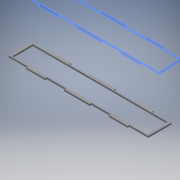
# Autodesk Inventor part: letreiro
Saved by Autodesk Inventor 2016 (Build 200138000, 138)
## iProperties
Created: 2017-06-07
Part Number: letreiro
Material: Generic
Document SubType Name: Modeling
Designer: fabio-note
Density: 1 g/cm^3
Appearance: Default
Author: fabio-note
Autodesk Inventor part; units mm, degrees
ref_plane "YZ Plane" through (0, 0, 0) normal (1, 0, 0) x (0, 1, 0)
ref_plane "XZ Plane" through (0, 0, 0) normal (0, 1, 0) x (-1, 0, 0)
ref_plane "XY Plane" through (0, 0, 0) normal (0, 0, 1) x (1, 0, 0)
sketch "Sketch1" plane through (0, 0, 0) normal (0, 0, 1) x (1, 0, 0)
  line L0 (-173, 32.5) -> (173, 32.5)
  line L1 (173, 32.5) -> (173, -32.5)
  line L2 (173, -32.5) -> (-173, -32.5)
  line L3 (-173, -32.5) -> (-173, 32.5)
  point P0 (0, 0)
  point P1 (173, 0)
  point P2 (0, 32.5)
  dimension "d0" = 65
  dimension "d1" = 346
  constraints: 8 end point, 2 midpoint, 2 parallel, 1 horizontal, 1 horizontal alignment, 1 perpendicular, 1 vertical alignment
  measures "d0" distance between parallel lines of L0 L2
  measures "d1" distance between parallel lines of L3 L1
extrude "Extrusion1" add sketch "Sketch1" along normal blind 4
sketch "Sketch2" plane through (0, 0, 4) normal (0, 0, 1) x (1, 0, 0)
  line L0 (-159, 25.5) -> (159, 25.5)
  line L1 (159, 25.5) -> (159, -25.5)
  line L2 (159, -25.5) -> (-159, -25.5)
  line L3 (-159, -25.5) -> (-159, 25.5)
  line L4 (173, 32.5) -> (-173, 32.5) projected
  line L5 (-173, 32.5) -> (-173, -32.5) projected
  line L6 (-173, -32.5) -> (173, -32.5) projected
  line L7 (173, -32.5) -> (173, 32.5) projected
  point P0 (0, 0)
  dimension "d4" = 7
  dimension "d5" = 14
  dimension "d6" = 7
  dimension "d7" = 14
  constraints: 8 end point, 2 parallel, 1 horizontal, 1 perpendicular
  measures "d4" distance between parallel lines of L4 L0
  measures "d5" distance between parallel lines of L5 L3
  measures "d6" distance between parallel lines of L6 L2
  measures "d7" distance between parallel lines of L7 L1
extrude "Extrusion2" cut sketch "Sketch2" against normal blind 10 contours L0 L1 L2 L3
sketch "Esboço3" plane through (0, 0, 4) normal (0, 0, 1) x (1, 0, 0)
  line L0 (-118.5, 32.5) -> (-118.5, 28.5)
  line L1 (-118.5, 28.5) -> (-165, 28.5)
  line L2 (-70.5, 32.5) -> (-24, 32.5)
  line L3 (-24, 32.5) -> (-24, 28.5)
  line L4 (-24, 28.5) -> (-70.5, 28.5)
  line L5 (-70.5, 28.5) -> (-70.5, 32.5)
  circle A0 centre (-118.5, 28.5) radius 1
  circle A1 centre (-70.5, 28.5) radius 1
  circle A2 centre (-24, 28.5) radius 1
  line L6 (-165, 28.5) -> (-165, 32.5)
  line L7 (-165, 32.5) -> (-118.5, 32.5)
  line L8 (173, 32.5) -> (-173, 32.5) projected
  line L9 (-173, 32.5) -> (-173, -32.5) projected
  circle A3 centre (-165, 28.5) radius 1
  point P0 (0, 0)
  dimension "d12" = 46.5
  dimension "d13" = 48
  dimension "d14" = 2
  dimension "d15" = 2
  dimension "d16" = 2
  dimension "d19" = 8
  dimension "d20" = 46.5
  dimension "d21" = 2
  constraints: 16 end point, 4 centre point, 4 coincident, 2 parallel, 1 collinear, 1 horizontal, 1 perpendicular, 1 vertical
  measures "d12" distance of L3.end L4.end
  measures "d13" distance between parallel lines of L0 L5
  measures "d14" diameter of A0
  measures "d15" diameter of A1
  measures "d16" diameter of A2
  measures "d19" distance between parallel lines of L9 L6
  measures "d20" distance between parallel lines of L0 L6
  measures "d21" diameter of A3
extrude "Extrusão3" cut sketch "Esboço3" against normal blind 10
mirror "Espelhamento1" about plane through (0, 0, 0) normal (1, 0, 0) of "Extrusão3"
mirror "Espelhamento2" about plane through (0, 0, 0) normal (0, 1, 0) of "Extrusão3", "Espelhamento1"
sketch "Esboço4" plane through (0, 0, 4) normal (0, 0, 1) x (1, 0, 0)
  line L0 (-173, 32.5) -> (-173, -32.5) projected
  line L1 (-173, -12.5) -> (-165, -12.5)
  line L2 (-165, -12.5) -> (-165, 12.5)
  line L3 (-165, 12.5) -> (-173, 12.5)
  line L4 (-173, 12.5) -> (-173, -12.5)
  line L5 (-165, 32.5) -> (-173, 32.5) projected
  line L6 (-173, -32.5) -> (-165, -32.5) projected
  circle A0 centre (-165, 12.5) radius 1
  circle A1 centre (-165, -12.5) radius 1
  point P0 (0, 0)
  dimension "d22" = 8
  dimension "d23" = 20
  dimension "d24" = 25
  dimension "d25" = 20
  dimension "d26" = 2
  dimension "d27" = 2
  constraints: 8 end point, 2 centre point, 2 coincident, 2 parallel, 1 horizontal, 1 perpendicular, 1 point on line
  measures "d22" distance of L3.end L2.end
  measures "d23" distance between parallel lines of L5 L3
  measures "d24" distance between parallel lines of L1 L3
  measures "d25" distance between parallel lines of L6 L1
  measures "d26" diameter of A0
  measures "d27" diameter of A1
extrude "Extrusão4" cut sketch "Esboço4" against normal blind 10
mirror "Espelhamento3" about plane through (0, 0, 0) normal (1, 0, 0) of "Extrusão4"
body "Solid1"
